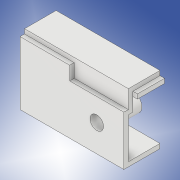
# Autodesk Inventor part: FA003
Saved by Autodesk Inventor 2017 SP1 (Build 210196100, 196)
## iProperties
Created: 2017-06-16
Part Number: FA003
Material: ABS Plastic
Document SubType Name: Modeling
Designer: Zach
Density: 1.06 g/cm^3
Appearance: CR White
Author: Zach
Autodesk Inventor part; units mm, degrees
ref_plane "YZ Plane" through (0, 0, 0) normal (1, 0, 0) x (0, 1, 0)
ref_plane "XZ Plane" through (0, 0, 0) normal (0, 1, 0) x (-1, 0, 0)
ref_plane "XY Plane" through (0, 0, 0) normal (0, 0, 1) x (1, 0, 0)
sketch "Sketch1" plane through (0, 0, 0) normal (0, 0, 1) x (1, 0, 0)
  line L0 (0, 0) -> (115, 0)
  line L1 (115, 0) -> (115, 75)
  line L2 (115, 75) -> (0, 75)
  line L3 (0, 75) -> (0, 0)
  dimension "d0" = 115
  dimension "d1" = 75
  constraints: 8 end point, 2 parallel, 1 horizontal, 1 perpendicular
  measures "d0" distance of L2.end L1.end
  measures "d1" distance of L1.end L0.end
extrude "Extrusion1" add sketch "Sketch1" along normal blind 40
sketch "Sketch2" plane through (0, 0, 40) normal (0, 0, 1) x (1, 0, 0)
  line L0 (115, 75) -> (0, 75) projected
  line L1 (115, 0) -> (115, 75) projected
  line L2 (0, 75) -> (115, 75)
  line L3 (115, 75) -> (115, 55)
  line L4 (115, 55) -> (0, 55)
  line L5 (0, 55) -> (0, 75)
  point P0 (0, 0)
  dimension "d4" = 20
  constraints: 8 end point, 2 parallel, 1 horizontal, 1 perpendicular, 1 point on line
  measures "d4" distance of L2.end L3.end
extrude "Extrusion2" cut sketch "Sketch2" against normal blind 5
sketch "Sketch3" plane through (115, 0, 0) normal (1, 0, 0) x (0, 0, -1)
  line L0 (0, 75) -> (-35, 75) projected
  line L1 (-35, 75) -> (-35, 55) projected
  line L2 (-35, 55) -> (-40, 55) projected
  line L3 (-40, 0) -> (-40, 55) projected
  line L4 (0, 0) -> (-40, 0) projected
  line L5 (0, 70) -> (-30, 70)
  line L6 (-30, 70) -> (-30, 50)
  line L7 (-30, 50) -> (-35, 50)
  line L8 (-35, 50) -> (-35, 5)
  line L9 (-35, 5) -> (0, 5)
  line L10 (0, 5) -> (0, 70)
  line L11 (0, 0) -> (0, 75) projected
  dimension "d7" = 5
  constraints: 12 end point, 1 collinear, 4 other
  measures "d7" distance between parallel lines of L0 L5
extrude "Extrusion3" cut sketch "Sketch3" against normal through all contours L10 L9 L8 L7 L6 L5
sketch "Sketch11" plane through (0, 0, 0) normal (0, 0, -1) x (-1, 0, 0)
  line L0 (-120, 70) -> (5, 70)
  line L1 (5, 70) -> (5, 65)
  line L2 (5, 65) -> (-120, 65)
  line L3 (-120, 65) -> (-120, 70)
  line L4 (-115, 70) -> (-115, 75) projected
  point P0 (0, 0)
  point P1 (0, 70)
  dimension "d42" = 5
  dimension "d43" = 5
  dimension "d44" = 5
  constraints: 8 end point, 2 parallel, 1 horizontal, 1 horizontal alignment, 1 perpendicular
  measures "d42" distance of L0.end L1.end
  measures "d43" distance between parallel lines of L4 L3
  measures "d44" distance from line of point (0, 70) L1
extrude "Extrusion10" add sketch "Sketch11" against normal blind 30
sketch "Sketch12" plane through (0, 0, 40) normal (0, 0, 1) x (1, 0, 0)
  circle A0 centre (85, 30) radius 7.5
  line L0 (0, 0) -> (115, 0) projected
  line L1 (115, 0) -> (115, 55) projected
  dimension "d47" = 15
  dimension "d48" = 30
  dimension "d49" = 30
  constraints: 1 centre point
  measures "d47" diameter of A0
  measures "d48" distance from line of L0 A0.centre
  measures "d49" distance from line of L1 A0.centre
extrude "Extrusion11" cut sketch "Sketch12" against normal through all
sketch "Sketch13" plane through (115, 5, 35) normal (0, 0, -1) x (-1, 0, 0)
  circle A0 centre (30, 25) radius 7.5 projected
  circle A1 centre (30, 25) radius 10
  point P0 (115, -5)
  dimension "d52" = 20
  constraints: 1 centre point, 1 coincident
  measures "d52" diameter of A1
extrude "Extrusion12" add sketch "Sketch13" along normal blind 35
sketch "Sketch14" plane through (85, 30, 0) normal (0, 0, -1) x (-1, 0, 0)
  circle A0 centre (0, 0) radius 7.5 projected
  circle A1 centre (0, 0) radius 2.5
  point P0 (85, -30)
  dimension "d55" = 5
  constraints: 1 centre point, 1 coincident
  measures "d55" diameter of A1
extrude "Extrusion13" add sketch "Sketch14" against normal blind 10
sketch "Sketch15" plane through (115, 5, 35) normal (0, 0, -1) x (-1, 0, 0)
  line L0 (115, 60) -> (0, 60) projected
  line L1 (0, 45) -> (115, 45) projected
  line L2 (115, 60) -> (65, 60)
  line L3 (65, 60) -> (65, 45)
  line L4 (65, 45) -> (115, 45)
  line L5 (115, 45) -> (115, 60)
  point P0 (115, -5)
  dimension "d58" = 50
  constraints: 8 end point, 2 parallel, 1 horizontal, 1 perpendicular, 1 point on line
  measures "d58" distance of L4.end L3.end
extrude "Extrusion14" cut sketch "Sketch15" along normal blind 10
sketch "Sketch16" plane through (0, 0, 35) normal (0, 0, 1) x (1, 0, 0)
  line L0 (0, 70) -> (0, 65) projected
  line L1 (55, 55) -> (0, 55)
  line L2 (0, 70) -> (55, 70)
  line L3 (55, 70) -> (55, 55)
  line L4 (55, 55) -> (0, 55)
  line L5 (0, 55) -> (0, 70)
  line L6 (50, 65) -> (50, 55) projected
  point P0 (0, 0)
  dimension "d63" = 5
  constraints: 10 end point, 2 parallel, 1 horizontal, 1 perpendicular
  measures "d63" distance between parallel lines of L3 L6
extrude "Extrusion15" add sketch "Sketch16" along normal blind 5
body "Solid1"
